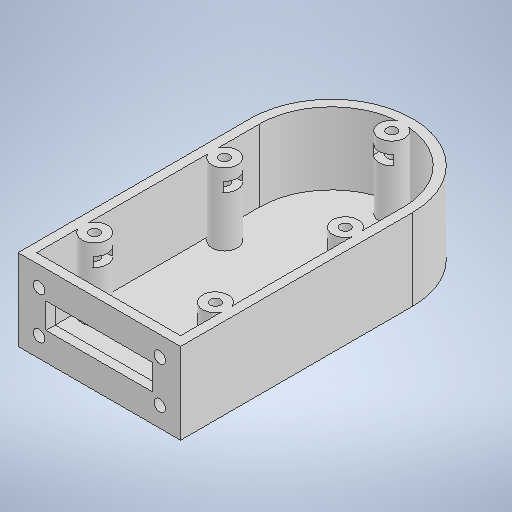
# Autodesk Inventor part: SCARA arm
Saved by Autodesk Inventor 2025.2 (Build 292293000, 293)
## iProperties
Created: 2025-01-27
Part Number: SCARA arm
Material: Generic
Document SubType Name: Modeling
Designer: caomi
Density: 1 g/cm^3
Appearance: Default
Author: caomi
Autodesk Inventor part; units mm, degrees
ref_plane "YZ Plane" through (0, 0, 0) normal (1, 0, 0) x (0, 1, 0)
ref_plane "XZ Plane" through (0, 0, 0) normal (0, 1, 0) x (-1, 0, 0)
ref_plane "XY Plane" through (0, 0, 0) normal (0, 0, 1) x (1, 0, 0)
sketch "Sketch1" plane through (0, 0, 0) normal (0, 1, 0) x (-1, 0, 0)
  line L0 (0, 0) -> (70, 0)
  line L1 (70, 0) -> (70, -100)
  line L2 (70, -100) -> (0, -100)
  line L3 (0, -100) -> (0, 0)
  circle A0 centre (35, -100) radius 35
  point P0 (0, -100)
  dimension "d0" = 70
  dimension "d1" = 100
  constraints: 8 end point, 2 parallel, 1 horizontal, 1 midpoint, 1 perpendicular, 3 other
  measures "d0" distance of L0.start L0.end
  measures "d1" distance between parallel lines of L2 L0
extrude "Extrusion1" add sketch "Sketch1" along normal blind 35
shell "Shell1" thickness 4 removed faces 1 at (-23.3333, 35, -33.3333)
sketch "Sketch2" plane through (-70, 0, 0) normal (0, 0, 1) x (1, 0, 0)
  line L0 (35, 44.7542) -> (35, -30.4775) construction
  line L1 (75.874, 17.5) -> (-5.874, 17.5) construction
  line L2 (0, 35) -> (70, 35) projected
  line L3 (70, 0) -> (70, 35) projected
  line L4 (0, 0) -> (0, 35) projected
  line L5 (0, 0) -> (70, 0) projected
  line L6 (58, 23) -> (12, 23)
  line L7 (12, 23) -> (12, 12)
  line L8 (12, 12) -> (58, 12)
  line L9 (58, 12) -> (58, 23)
  circle A0 centre (9, 26.5) radius 2.5
  circle A1 centre (61, 8.5) radius 2.5
  circle A2 centre (9, 8.5) radius 2.5
  circle A3 centre (61, 26.5) radius 2.5
  point P0 (35, 17.5)
  point P1 (35, 35)
  point P2 (70, 17.5)
  dimension "d7" = 12
  dimension "d8" = 5
  dimension "d9" = 52
  dimension "d10" = 18
  constraints: 12 end point, 4 centre point, 3 midpoint, 3 point on line, 1 equal radius, 1 horizontal, 1 symmetric about line, 1 vertical, 5 other
  measures "d7" distance between parallel lines of L2 L6
  measures "d8" diameter of A1
  measures "d9" distance of A1.centre A2.centre
  measures "d10" distance of A3.centre A1.centre
extrude "Extrusion2" cut sketch "Sketch2" against normal blind 52 contours L9 L8 L7 L6 | A0 | A1 | A2 | A3
sketch "Sketch3" plane through (0, 35, 0) normal (0, 1, 0) x (1, 0, 0)
  circle A0 centre (-61, 24) radius 2.15
  line L0 (-63.396, 28.15) -> (-58.604, 28.15)
  line L1 (-58.604, 28.15) -> (-56.208, 24)
  line L2 (-56.208, 24) -> (-58.604, 19.85)
  line L3 (-58.604, 19.85) -> (-63.396, 19.85)
  line L4 (-63.396, 19.85) -> (-65.792, 24)
  line L5 (-65.792, 24) -> (-63.396, 28.15)
  circle A1 centre (-61, 24) radius 5.5
  line L6 (-58.604, 19.85) -> (-57.3906, 19.85)
  line L7 (-58.604, 28.15) -> (-57.3906, 28.15)
  line L8 (-66, 4) -> (-66, 100) projected
  line L9 (-4, 4) -> (-66, 4) projected
  line L10 (23.6723, 52) -> (-94.1512, 52) construction
  line L11 (-35, -9.527) -> (-35, 93.21) construction
  circle A2 centre (-61, 80) radius 2.15
  line L12 (-63.396, 75.85) -> (-58.604, 75.85)
  line L13 (-58.604, 75.85) -> (-56.208, 80)
  line L14 (-56.208, 80) -> (-58.604, 84.15)
  line L15 (-58.604, 84.15) -> (-63.396, 84.15)
  line L16 (-63.396, 84.15) -> (-65.792, 80)
  line L17 (-65.792, 80) -> (-63.396, 75.85)
  circle A3 centre (-61, 80) radius 5.5
  line L18 (-58.604, 84.15) -> (-57.3906, 84.15)
  line L19 (-58.604, 75.85) -> (-57.3906, 75.85)
  circle A4 centre (-9, 24) radius 2.15
  line L20 (-6.604, 28.15) -> (-11.396, 28.15)
  line L21 (-11.396, 28.15) -> (-13.792, 24)
  line L22 (-13.792, 24) -> (-11.396, 19.85)
  line L23 (-11.396, 19.85) -> (-6.604, 19.85)
  line L24 (-6.604, 19.85) -> (-4.208, 24)
  line L25 (-4.208, 24) -> (-6.604, 28.15)
  circle A5 centre (-9, 24) radius 5.5
  line L26 (-11.396, 19.85) -> (-12.6094, 19.85)
  line L27 (-11.396, 28.15) -> (-12.6094, 28.15)
  line L28 (-11.396, 75.85) -> (-12.6094, 75.85)
  line L29 (-11.396, 75.85) -> (-13.792, 80)
  circle A6 centre (-9, 80) radius 2.15
  line L30 (-11.396, 84.15) -> (-12.6094, 84.15)
  line L31 (-13.792, 80) -> (-11.396, 84.15)
  line L32 (-6.604, 75.85) -> (-11.396, 75.85)
  line L33 (-11.396, 84.15) -> (-6.604, 84.15)
  line L34 (-4.208, 80) -> (-6.604, 75.85)
  line L35 (-6.604, 84.15) -> (-4.208, 80)
  circle A7 centre (-9, 80) radius 5.5
  circle A8 centre (-35, 126) radius 2.15
  line L36 (-39.15, 123.604) -> (-39.15, 128.396)
  line L37 (-39.15, 128.396) -> (-35, 130.792)
  line L38 (-35, 130.792) -> (-30.85, 128.396)
  line L39 (-30.85, 128.396) -> (-30.85, 123.604)
  line L40 (-30.85, 123.604) -> (-35, 121.208)
  line L41 (-35, 121.208) -> (-39.15, 123.604)
  circle A9 centre (-35, 126) radius 5.5
  arc A10 (-4, 100) -> (-66, 100) centre (-35, 100) ccw projected
  line L42 (-39.15, 123.604) -> (-39.15, 122.3906)
  line L43 (-30.85, 123.604) -> (-30.85, 122.3906)
  point P0 (0, 0)
  point P1 (-35, 4)
  point P2 (-66, 52)
  point P3 (-35, 131)
  point P4 (-32.5001, 130.899)
  point P5 (-37.4999, 130.899)
  dimension "d14" = 4.3
  dimension "d15" = 11
  dimension "d16" = 8.3
  dimension "d19" = 5
  dimension "d20" = 20
  dimension "d21" = 4.3
  dimension "d22" = 8.3
  dimension "d23" = 11
  dimension "d24" = 5
  constraints: 84 end point, 32 symmetric about line, 11 point on circle, 10 centre point, 8 coincident, 4 horizontal, 4 point on line, 2 midpoint, 2 vertical, 1 parallel, 32 other
  measures "d14" diameter of A0
  measures "d15" diameter of A1
  measures "d16" distance between parallel lines of L0 L3
  measures "d19" distance from line of A0.centre L8
  measures "d20" distance from line of L9 A0.centre
  measures "d21" diameter of A8
  measures "d22" distance between parallel lines of L39 L36
  measures "d23" diameter of A9
  measures "d24" distance of point (-35, 131) A8.centre
extrude "Extrusion3" add sketch "Sketch3" against normal up to surface (31 mm away) contours L5 L4 L3 L6 A1 L8 L7 L0 | L0 L1 L2 L3 L4 L5 | L7 A1 L6 L2 L1 | L8 A1 | A3 L8 | L8 A3 L18 L15 L16 L17 L12 L19 | L19 L13 L14 L18 A3 | L12 L17 L16 L15 L14 L13 | L25 L24 L23 L22 L21 L20 | L20 L27 A5 L26 L23 L24 L25 | L21 L22 L26 A5 L27 | L32 L34 L35 L33 L30 A7 L28 | L28 A7 L30 L31 L29 | L29 L31 L33 L35 L34 L32 | L42 A9 A10 L43 L39 L38 L37 L36 | L36 L37 L38 L39 L40 L41 | L41 L40 L43 A9 L42
ref_plane "Work Plane1" through (0, 30, 0) normal (0, 1, 0) x (1, 0, 0)
extrude "Extrusion4" cut sketch "Sketch3" against normal blind 4.2 from surface at -5 contours L0 L1 L2 L3 L4 L5 | L7 A1 L6 L2 L1 | L19 L13 L14 L18 A3 | L12 L17 L16 L15 L14 L13 | L25 L24 L23 L22 L21 L20 | L21 L22 L26 A5 L27 | L28 A7 L30 L31 L29 | L29 L31 L33 L35 L34 L32 | L36 L37 L38 L39 L40 L41 | L41 L40 L43 A9 L42
equation "\"d11\" = d9"
equation "\"d21\" = d14"
equation "\"d22\" = d16"
equation "\"d23\" = d15"
body "Solid1"
